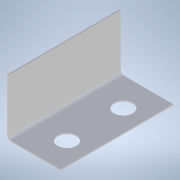
# Autodesk Inventor part: Clmap for sample mount for new Leica System
Saved by Autodesk Inventor 2020.5 (Build 245400000, 400)
## iProperties
Created: 2022-08-03
Part Number: Clmap for sample mount for new Leica System
Material: Generic
Document SubType Name: Modeling
Designer: Julian
Density: 1 g/cm^3
Appearance: Default
Author: Julian
Autodesk Inventor part; units mm, degrees
ref_plane "YZ Plane" through (0, 0, 0) normal (1, 0, 0) x (0, 1, 0)
ref_plane "XZ Plane" through (0, 0, 0) normal (0, 1, 0) x (-1, 0, 0)
ref_plane "XY Plane" through (0, 0, 0) normal (0, 0, 1) x (1, 0, 0)
sketch "Sketch1" plane through (0, 0, 0) normal (0, 1, 0) x (-1, 0, 0)
  line L0 (0, 0) -> (11.5, 0)
  line L1 (11.5, 0) -> (11.5, -12)
  line L2 (11.5, -12) -> (0, -12)
  line L3 (0, -12) -> (0, 0)
  line L4 (0, -12) -> (5.2, -12)
  line L5 (5.2, -12) -> (5.2, 0)
  line L6 (5.2, 0) -> (0, 0)
  line L7 (0, 0) -> (0, -12)
  line L8 (0, 0) -> (2.3, 0)
  line L9 (2.3, 0) -> (2.3, -12)
  line L10 (2.3, -12) -> (0, -12)
  line L11 (0, -12) -> (0, 0)
  line L12 (2.3, 0) -> (2.3, -3)
  line L13 (2.3, -3) -> (2.3, -9)
  circle A0 centre (2.3, -3) radius 1
  circle A1 centre (2.3, -9) radius 1
  dimension "d0" = 11.5
  dimension "d1" = 12
  dimension "d2" = 5.2
  dimension "d3" = 2.3
  dimension "d4" = 3
  dimension "d5" = 6
  dimension "d6" = 2
  dimension "d7" = 2
  constraints: 28 end point, 6 parallel, 4 point on line, 3 horizontal, 3 perpendicular, 2 centre point, 2 coincident
  measures "d0" distance of L1.end L2.end
  measures "d1" distance of L0.end L1.end
  measures "d2" distance of L6.end L5.end
  measures "d3" distance of L9.end L10.end
  measures "d4" distance of L8.end L12.end
  measures "d5" distance of L12.end L13.end
  measures "d6" diameter of A0
  measures "d7" diameter of A1
extrude "Extrusion1" add sketch "Sketch1" along normal blind 0.13 contours L0 L9 A0 A1 L2 L3 | L0 L5 L2 L9 A1 A0 | L0 L1 L2 L5
bend part "Bend Part1" radius 0.5 angle 90 line through (-5.2, 0, -12) along (0, 0, 1) centre toward (0, 1, 0) moving side (-1, 0, 0) both sides no
body "Solid1"
